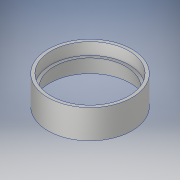
# Autodesk Inventor part: Aluminum Skirt
Saved by Autodesk Inventor 2017 (Build 210142000, 142)
## iProperties
Created: 2016-07-25
Part Number: Aluminum Skirt
Material: Aluminum 6061
Document SubType Name: Modeling
Designer: Jared
Density: 2.7 g/cm^3
Appearance: Aluminum - Flat
Author: Jared
Autodesk Inventor part; units mm, degrees
ref_plane "YZ Plane" through (0, 0, 0) normal (1, 0, 0) x (0, 1, 0)
ref_plane "XZ Plane" through (0, 0, 0) normal (0, 1, 0) x (-1, 0, 0)
ref_plane "XY Plane" through (0, 0, 0) normal (0, 0, 1) x (1, 0, 0)
sketch "Sketch1" plane through (0, 0, 0) normal (0, 0, 1) x (1, 0, 0)
  line L0 (0, 25.4) -> (-28.702, 25.4) construction
  line L1 (0, 25.4) -> (-95.25, 25.4) construction
  line L2 (-95.25, 25.4) -> (-88.9, 25.4) construction
  line L3 (-88.9, 25.4) -> (-82.55, 22.4389) construction
  line L4 (-88.9, 25.4) -> (-88.9, 22.4389) construction
  line L5 (-88.9, 0) -> (-95.25, 0)
  line L6 (-28.702, 59.6457) -> (-28.702, -91.9304) construction
  arc A0 (-28.9184, -8.3597) -> (-32.3684, -0.9611) centre (-35.052, -6.7162) ccw
  line L7 (-76.2, -184.8171) -> (-28.702, -7.5522)
  line L8 (-88.9, 22.4389) -> (-82.55, 22.4389)
  line L9 (-88.9, 22.4389) -> (-88.9, 0)
  line L10 (-82.55, 22.4389) -> (-32.3684, -0.9611)
  line L11 (-28.702, -6.7162) -> (-60.452, -6.7162) construction
  line L12 (-60.452, 12.1345) -> (-60.452, -126.0448) construction
  line L13 (-60.452, -126.0448) -> (-54.102, -126.0448) construction
  line L14 (-54.102, -126.0448) -> (-54.102, -102.3463) construction
  line L15 (-54.102, -102.3463) -> (-60.452, -102.3463)
  line L16 (-60.452, 12.1345) -> (-60.452, 2.6095) construction
  line L17 (-60.452, 12.1345) -> (-60.452, 5.7845) construction
  line L18 (-60.452, 5.7845) -> (-46.8344, 5.7845)
  line L19 (-60.452, 5.7845) -> (-60.452, -102.3463)
  line L20 (-95.25, 0) -> (-95.25, -12.7) construction
  line L21 (-60.452, -12.7) -> (-73.152, -12.7) construction
  line L22 (-95.25, -12.7) -> (-95.25, -25.4) construction
  line L23 (-95.25, -25.4) -> (-95.25, -88.9) construction
  line L24 (-95.25, -88.9) -> (-82.55, -88.9) construction
  line L25 (-82.55, -88.9) -> (-82.55, -25.4) construction
  line L26 (-95.25, -25.4) -> (-82.55, -25.4)
  line L27 (-82.55, -25.4) -> (-82.55, -88.9)
  line L28 (-82.55, -88.9) -> (-95.25, -88.9)
  line L29 (-95.25, -12.7) -> (-73.152, -12.7)
  line L30 (-73.152, -137.8941) -> (-63.627, -137.8941)
  line L31 (-82.55, -88.9) -> (-82.55, -184.8171)
  line L32 (-82.55, -184.8171) -> (-76.2, -184.8171)
  line L33 (-73.152, -12.7) -> (-73.152, -137.8941)
  line L34 (-88.9, -25.4) -> (-88.9, -31.3436)
  line L35 (-88.9, -31.3436) -> (-95.25, -31.3436)
  line L36 (-95.25, 0) -> (-95.25, -25.4)
  line L37 (-95.25, -31.3436) -> (-95.25, -88.9)
  line L38 (-88.9, -159.4171) -> (-88.9, -220.3649)
  line L39 (-28.9184, -8.3597) -> (-85.725, -220.3649)
  line L40 (-85.725, -220.3649) -> (-88.9, -220.3649)
  line L41 (-82.55, -159.4171) -> (-88.9, -159.4171)
  line L42 (0, -319.0244) -> (0, 122.7573) projected
  point P0 (0, 0)
  point P1 (-95.25, -255.9127)
  point P2 (-85.725, 22.4389)
  dimension "d0" = 28.702
  dimension "d1" = 95.25
  dimension "d2" = 6.35
  dimension "d3" = 25
  dimension "d5" = 25.4
  dimension "d6" = 25.4
  dimension "d8" = 12.7
  dimension "d11" = 6.35
  dimension "d12" = 31.75
  dimension "d13" = 6.35
  dimension "d15" = 6.35
  dimension "d16" = 12.7
  dimension "d17" = 12.7
  dimension "d18" = 12.7
  dimension "d19" = 63.5
  dimension "d20" = 12.7
  dimension "d22" = 9.525
  dimension "d23" = 6.35
  dimension "d25" = 5.9436
  dimension "d26" = 15
  dimension "d27" = 3.175
  dimension "d28" = 6.35
  dimension "d29" = 25.4
  constraints: 84 end point, 18 point on line, 17 perpendicular, 12 vertical, 5 horizontal, 5 tangent, 5 vertical alignment, 3 midpoint, 3 point on circle, 2 collinear, 1 centre point
  measures "d0" distance of L0.start L0.end
  measures "d1" distance of L0.start L1.end
  measures "d2" distance of L1.end L2.end
  measures "d3" angle of L1 L3
  measures "d5" distance of point (0, 0) L0.start
  measures "d6" distance of L2.end L5.start
  measures "d8" diameter of A0
  measures "d11" distance of L4.end L3.end
  measures "d12" distance of L11.start L11.end
  measures "d13" distance of L12.end L13.end
  measures "d15" distance of L12.start L17.end
  measures "d16" distance of L5.end L20.end
  measures "d17" distance of L21.start L21.end
  measures "d18" distance of L20.end L22.end
  measures "d19" distance of L23.end L22.end
  measures "d20" distance of L23.end L24.end
  measures "d22" distance of L30.start L30.end
  measures "d23" distance of L31.end L7.start
  measures "d25" distance of L34.start L34.end
  measures "d26" angle of L7 L19
  measures "d27" distance of L38.end L39.end
  measures "d28" distance of L41.start L38.start
  measures "d29" distance from line of L31.end L41
revolve "Revolution1" add sketch "Sketch1" angle 360 about axis through (0, -10, 0) along (0, 1, 0) contours L39 L40 L38 L41 L31 L32
body "Solid1"
